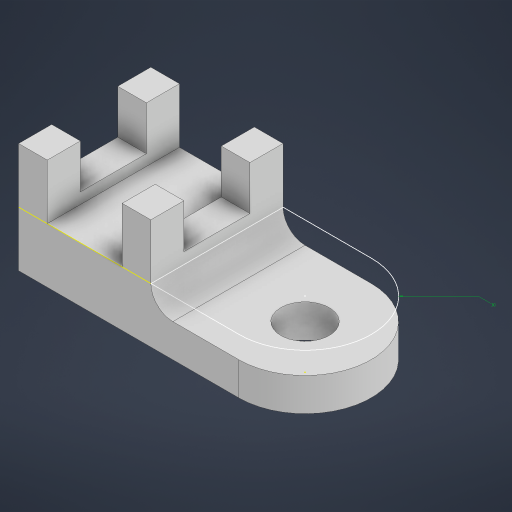
# Autodesk Inventor part: Part3
Saved by Autodesk Inventor 2023 (Build 270158000, 158)
## iProperties
Created: 2023-04-25
Part Number: Part3
Material: Ogólny
Document SubType Name: Modeling
Designer: Adam
Density: 1 g/cm^3
Appearance: Domyślna
Author: Adam
Autodesk Inventor part; units mm, degrees
ref_plane "YZ Plane" through (0, 0, 0) normal (1, 0, 0) x (0, 1, 0)
ref_plane "XZ Plane" through (0, 0, 0) normal (0, 1, 0) x (-1, 0, 0)
ref_plane "XY Plane" through (0, 0, 0) normal (0, 0, 1) x (1, 0, 0)
sketch "Szkic1" plane through (0, 0, 0) normal (0, 1, 0) x (-1, 0, 0)
  line L0 (130, 0) -> (30, 0)
  line L1 (0, -30) -> (0, -30)
  line L2 (30, -60) -> (130, -60)
  line L3 (130, -60) -> (130, 0)
  arc A0 (30, 0) -> (0, -30) centre (30, -30) ccw
  arc A1 (0, -30) -> (30, -60) centre (30, -30) ccw
  point P0 (0, 0)
  point P1 (0, -60)
  point P2 (0, 0)
  dimension "d0" = 130
  dimension "d1" = 60
  dimension "d2" = 30
  constraints: 8 end point, 4 point on circle, 4 point on line, 4 tangent, 2 centre point, 2 parallel, 1 coincident, 1 concentric, 1 horizontal, 1 perpendicular
  measures "d0" distance of point (0, -60) L2.end
  measures "d1" distance of L2.end L0.start
  measures "d2" radius of A0
extrude "Wyciągnięcie proste1" add sketch "Szkic1" along normal blind 25
sketch "Szkic2" plane through (0, 25, 0) normal (0, 1, 0) x (1, 0, 0)
  arc A0 (-30, 0) -> (-30, 60) centre (-30, 30) ccw projected
  point P0 (0, 0)
  constraints: 1 coincident
hole "Otwór1" at (-30, 25, -30) direction (0, -1, 0) diameter 22 end through all
sketch "Szkic3" plane through (0, 25, 0) normal (0, 1, 0) x (1, 0, 0)
  line L0 (-30, 60) -> (-130, 60) projected
  line L1 (-130, 60) -> (-70, 60)
  line L2 (-70, 60) -> (-70, 0)
  line L3 (-70, 0) -> (-130, 0)
  line L4 (-130, 0) -> (-130, 60)
  point P0 (0, 0)
  dimension "d12" = 60
  dimension "d13" = 60
  dimension "d32" = 0
  dimension "d33" = 0
  constraints: 8 end point, 2 parallel, 1 horizontal, 1 perpendicular
  measures "d12" distance of L2.end L3.end
  measures "d13" distance of L1.end L2.end
  measures "d32" distance from line of point (-70, 60) L0
  measures "d33" distance from line of point (-70, 60) L2
extrude "Wyciągnięcie proste2" add sketch "Szkic3" along normal blind 25
sketch "Szkic4" plane through (0, 50, 0) normal (0, 1, 0) x (1, 0, 0)
  line L0 (-130, 60) -> (-130, 0) projected
  line L1 (-70, 0) -> (-70, 60) projected
  line L2 (-130, 45) -> (-70, 45)
  line L3 (-70, 45) -> (-70, 15)
  line L4 (-70, 15) -> (-130, 15)
  line L5 (-130, 15) -> (-130, 45)
  line L6 (-70, 60) -> (-130, 60) projected
  point P0 (0, 0)
  dimension "d16" = 15
  dimension "d17" = 30
  dimension "d28" = 15
  dimension "d29" = 0
  dimension "d30" = 45
  dimension "d31" = 60
  constraints: 8 end point, 2 parallel, 2 point on line, 1 horizontal, 1 perpendicular
  measures "d16" distance between parallel lines of L2 L6
  measures "d17" distance between parallel lines of L2 L4
  measures "d28" distance from line of point (-70, 45) L6
  measures "d29" distance from line of point (-70, 45) L1
  measures "d30" distance from line of point (-130, 15) L6
  measures "d31" distance from line of point (-130, 15) L1
extrude "Wyciągnięcie proste3" cut sketch "Szkic4" against normal blind 20 contours L2 L1 L4 L0
sketch "Szkic5" plane through (0, 50, 0) normal (0, 1, 0) x (1, 0, 0)
  line L0 (-70, 60) -> (-130, 60) projected
  line L1 (-130, 0) -> (-70, 0) projected
  line L2 (-117, 60) -> (-83, 60)
  line L3 (-83, 60) -> (-83, 0)
  line L4 (-83, 0) -> (-117, 0)
  line L5 (-117, 0) -> (-117, 60)
  line L6 (-70, 45) -> (-70, 60) projected
  point P0 (0, 0)
  dimension "d20" = 13
  dimension "d21" = 34
  constraints: 8 end point, 2 parallel, 2 point on line, 1 horizontal, 1 perpendicular
  measures "d20" distance between parallel lines of L3 L6
  measures "d21" distance between parallel lines of L3 L5
extrude "Wyciągnięcie proste4" cut sketch "Szkic5" against normal blind 25
sketch "Szkic6" plane through (0, 25, 0) normal (0, 1, 0) x (1, 0, 0)
  point P0 (0, 0)
sketch "Szkic7" plane through (0, 25, 0) normal (0, 1, 0) x (1, 0, 0)
  line L0 (-70, 45) -> (-70, 60) projected
  line L1 (-70, 60) -> (-70, 0)
  line L2 (-70, 0) -> (-30, 0)
  line L3 (-130, 0) -> (-30, 0) projected
  line L4 (0, 30) -> (0, 30)
  line L5 (-30, 60) -> (-70, 60)
  arc A0 (0, 30) -> (-30, 60) centre (-30, 30) ccw
  arc A1 (-30, 0) -> (0, 30) centre (-30, 30) ccw
  point P0 (0, 0)
  dimension "d24" = 30
  constraints: 8 end point, 4 point on circle, 4 tangent, 2 centre point, 2 collinear, 2 perpendicular, 2 point on line, 1 concentric
  measures "d24" radius of A0
extrude "Wyciągnięcie proste5" cut sketch "Szkic7" against normal blind 10
fillet "Zaokrąglenie powierzchni1" radius 10 1 edges at (-70, 15, -30)
